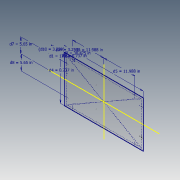
# Autodesk Inventor part: FLUGGER BACK COVER
Saved by Autodesk Inventor 2020.3 (Build 243373000, 373)
## iProperties
RuleStatus: InUse
AfterDocSave0: file://Part Number Cleaner
Created: 2020-01-03
Material: ACRYLIC, CLEAR
Vendor: HHMI: JRC - ID&F
Document SubType Name: Modeling
Designer: arnoldj
Density: 0.66 g/cm^3
Appearance: Clear - Light
DESIGN DEPARTMENT: HHMI: JRC - ID&F
ALTERED ITEM PART NUMBER: N/A
ALTERED ITEM VENDOR: N/A
ALTERED ITEM DESCRIPTION: N/A
Author: arnoldj
Revision Number: 0
Autodesk Inventor part; units mm, degrees
ref_plane "YZ Plane" through (0, 0, 0) normal (1, 0, 0) x (0, 1, 0)
ref_plane "XZ Plane" through (0, 0, 0) normal (0, 1, 0) x (-1, 0, 0)
ref_plane "XY Plane" through (0, 0, 0) normal (0, 0, 1) x (1, 0, 0)
sketch "Sketch1" plane through (0, 0, 0) normal (0, 0, 1) x (1, 0, 0)
  line L0 (0, 316.484) -> (0, -316.484) projected
  line L1 (-541.8455, 0) -> (541.8455, 0) projected
  line L2 (387.0325, -226.06) -> (-387.0325, -226.06)
  line L3 (-387.0325, -226.06) -> (-387.0325, 226.06)
  line L4 (-387.0325, 226.06) -> (387.0325, 226.06)
  line L5 (387.0325, 226.06) -> (387.0325, -226.06)
  line L6 (387.0325, -226.06) -> (-387.0325, 226.06) construction
  line L7 (-387.0325, -226.06) -> (387.0325, 226.06) construction
  line L8 (368.3127, -207.3402) -> (-368.3127, -207.3402) construction
  line L9 (-368.3127, -207.3402) -> (-368.3127, 207.3402) construction
  line L10 (-368.3127, 207.3402) -> (368.3127, 207.3402) construction
  line L11 (368.3127, 207.3402) -> (368.3127, -207.3402) construction
  line L12 (368.3127, -207.3402) -> (-368.3127, 207.3402) construction
  line L13 (-368.3127, -207.3402) -> (368.3127, 207.3402) construction
  point P0 (0, 0)
  point P1 (-304.4952, 207.3402)
  point P2 (0, 207.3402)
  point P3 (304.4952, 207.3402)
  point P4 (-304.4952, -207.3402)
  point P5 (0, -207.3402)
  point P6 (304.4952, -207.3402)
  point P7 (-368.3127, 143.51)
  point P8 (-368.3127, -143.51)
  point P9 (368.3127, 143.51)
  point P10 (368.3127, -117.0967)
  dimension "d0" = 774.065
  dimension "d1" = 452.12
  dimension "d3" = 18.7198
  dimension "d4" = 18.7198
  dimension "d5" = 304.4952
  dimension "d6" = 304.4952
  dimension "d7" = 143.51
  dimension "d8" = 143.51
  dimension "d9" = 82.5373
  dimension "d10" = 82.55
  constraints: 24 end point, 8 point on line, 6 midpoint, 4 parallel, 2 horizontal, 2 perpendicular, 2 vertical alignment, 1 horizontal alignment
  measures "d0" distance of L3.end L4.end
  measures "d1" distance of L2.end L3.end
  measures "d3" distance between parallel lines of L10 L4
  measures "d4" distance between parallel lines of L9 L3
  measures "d5" distance from line of L0 point (304.495, 207.34)
  measures "d6" distance from line of L0 point (-304.495, 207.34)
  measures "d7" distance from line of L1 point (-368.313, 143.51)
  measures "d8" distance from line of point (-368.313, -143.51) L1
  measures "d9" distance from line of point (-304.495, 207.34) L3
  measures "d10" distance from line of point (-368.313, 143.51) L4
extrude "Extrusion1" add sketch "Sketch1" against normal blind 4.4958
hole "Hole1" at (-304.4952, 207.3402, 0) at (0, 207.3402, 0) at (304.4952, 207.3402, 0) at (-304.4952, -207.3402, 0) at (0, -207.3402, 0) at (304.4952, -207.3402, 0) at (-368.3127, 143.51, 0) at (-368.3127, -143.51, 0) at (368.3127, 143.51, 0) at (368.3127, -117.0967, 0) direction (0, 0, -1) diameter 7.9375 end through all
fillet "Fillet1" radius 6.35 4 edges at (387.0325, 226.06, -2.2479) (387.0325, -226.06, -2.2479) (-387.0325, -226.06, -2.2479) (-387.0325, 226.06, -2.2479)
sketch "Sketch2" plane through (0, 0, 0) normal (0, 0, 1) x (1, 0, 0)
  line L0 (0, 316.484) -> (0, -316.484) projected
  line L1 (-541.8455, 0) -> (541.8455, 0) projected
  point P0 (0, 0)
  point P1 (-76.2, 101.6)
  point P2 (-76.2, 0)
  point P3 (-76.2, -101.6)
  dimension "d21" = 76.2
  dimension "d22" = 101.6
  dimension "d24" = 0
  dimension "d25" = 101.6
  measures "d21" distance from line of L0 point (-76.2, 101.6)
  measures "d22" distance from line of L1 point (-76.2, 101.6)
  measures "d24" distance from line of L1 point (-76.2, 0)
  measures "d25" distance from line of L1 point (-76.2, -101.6)
hole "Hole2" at (-76.2, 101.6, 0) at (-76.2, 0, 0) at (-76.2, -101.6, 0) direction (0, 0, -1) diameter 3.1242 end through all
body "Solid1"
